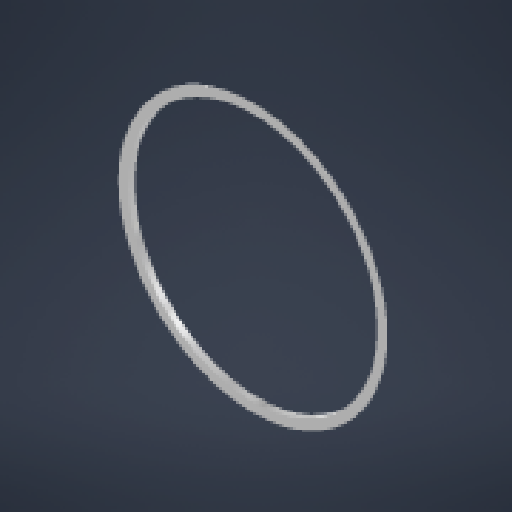
# Autodesk Inventor part: Support Ring, L-Section
Saved by Autodesk Inventor 2026 (Build 300175000, 175)
## iProperties
Created: 2025-11-02
Part Number: Support Ring, L-Section
Material: Aluminum 6061
Document SubType Name: Modeling
Designer: Brandon Portillo
Density: 2.7 g/cm^3
Appearance: Aluminum - Flat
Author: Brandon Portillo
Autodesk Inventor part; units mm, degrees
ref_plane "YZ Plane" through (0, 0, 0) normal (1, 0, 0) x (0, 1, 0)
ref_plane "XZ Plane" through (0, 0, 0) normal (0, 1, 0) x (-1, 0, 0)
ref_plane "XY Plane" through (0, 0, 0) normal (0, 0, 1) x (1, 0, 0)
sketch "Sketch1" plane through (0, 0, 0) normal (0, 1, 0) x (-1, 0, 0)
  line L0 (0, 0) -> (150, 0)
  line L1 (150, 0) -> (150, -6)
  line L2 (150, -6) -> (6, -6)
  line L3 (0, -6) -> (0, 0)
  line L4 (0, 0) -> (6, 0)
  line L5 (6, -6) -> (6, -100)
  line L6 (6, -100) -> (0, -100)
  line L7 (0, -100) -> (0, 0)
  line L8 (150, -3) -> (-2050, -3)
  line L9 (-2050, -3) -> (-2050, -100)
  dimension "d0" = 150
  dimension "d1" = 6
  dimension "d2" = 6
  dimension "d3" = 100
  dimension "d4" = 2200
  constraints: 20 end point, 4 parallel, 3 horizontal, 3 perpendicular, 1 midpoint
  measures "d0" distance of L1.end L3.start
  measures "d1" distance of L0.end L1.end
  measures "d2" distance of L5.end L6.end
  measures "d3" distance of L4.end L5.end
  measures "d4" distance of L8.start L8.end
revolve "Revolution1" add sketch "Sketch1" angle 360 about axis through (2050, 0, -3) along (0, 0, -1)
body "Solid1"
